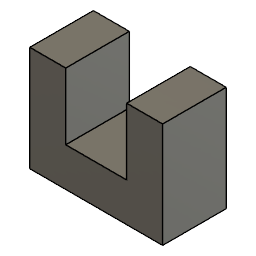
replay (Autodesk Fusion 360 design; units mm, degrees)
Autodesk Fusion 360 part; units mm, degrees
sketch "草图1" plane through (0, 0, 0) normal (0, 0, 1) x (1, 0, 0)
  line L0 (7, 44) -> (7, 6)
  line L1 (7, 6) -> (55, 6)
  line L2 (55, 6) -> (55, 44)
  line L3 (55, 44) -> (42, 44)
  line L4 (42, 44) -> (42, 20)
  line L5 (42, 20) -> (20, 20)
  line L6 (20, 20) -> (20, 44)
  line L7 (20, 44) -> (7, 44)
extrude "拉伸1" add sketch "草图1" along normal blind 23
